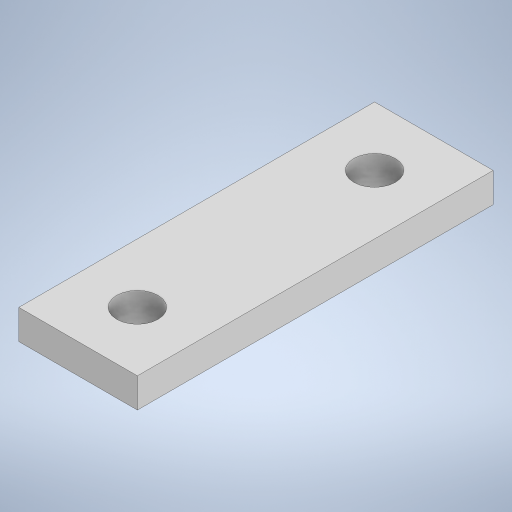
# Autodesk Inventor part: standard_union
Saved by Autodesk Inventor 2023 (Build 270158000, 158)
## iProperties
Created: 2022-12-26
Part Number: standard_union
Material: Genérico
Document SubType Name: Modeling
Designer: inigo
Density: 1 g/cm^3
Appearance: Valor por defecto
Author: inigo
Autodesk Inventor part; units mm, degrees
ref_plane "YZ Plane" through (0, 0, 0) normal (1, 0, 0) x (0, 1, 0)
ref_plane "XZ Plane" through (0, 0, 0) normal (0, 1, 0) x (-1, 0, 0)
ref_plane "XY Plane" through (0, 0, 0) normal (0, 0, 1) x (1, 0, 0)
sketch "Boceto1" plane through (0, 0, 0) normal (0, 1, 0) x (-1, 0, 0)
  circle A0 centre (0, 10) radius 1.75
  circle A1 centre (0, -10) radius 1.75
  line L0 (0, 10) -> (0, -10)
  line L1 (5, 15) -> (-5, 15)
  line L2 (-5, 15) -> (-5, -15)
  line L3 (-5, -15) -> (5, -15)
  line L4 (5, -15) -> (5, 15)
  line L5 (5, 15) -> (-5, -15) construction
  line L6 (-5, 15) -> (5, -15) construction
  point P0 (0, 0)
  point P1 (0, 0)
  constraints: 14 end point, 2 centre point
extrude "Extrusión1" add sketch "Boceto1" along normal blind 2.5
